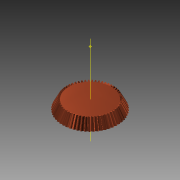
# Autodesk Inventor part: Bevel Gear2
Saved by Autodesk Inventor 2015 (Build 190141000, 141)
## iProperties
Created: 2008-07-23
Part Number: Bevel Gear2
Material: Steel, Mild
Document SubType Name: Modeling
Designer: tangg
Categories: <?xml version="1.0" encoding="UTF-16"?> <MemberInstance><Categories><FamilyTemplate><FamilyTemplateParameter ValueType="xs:double" Id="1" ObjectReferenceKey="da_z" ObjectType="kUserParameterObject"/><FamilyTemplateParameter ValueType="xs:double" Id="2" ObjectReferenceKey="da_b" ObjectType="kUserParameterObject"/><FamilyTemplateParameter ValueType="xs:double" Id="3" ObjectReferenceKey="da_beta" ObjectType="kUserParameterObject"/><FamilyTemplateParameter ValueType="xs:double" Id="4" ObjectReferenceKey="da_dae" ObjectType="kUserParameterObject"/><FamilyTemplateParameter ValueType="xs:double" Id="5" ObjectReferenceKey="da_ve" ObjectType="kUserParameterObject"/><FamilyTemplateParameter ValueType="xs:double" Id="6" ObjectReferenceKey="da_omega" ObjectType="kUserParameterObject"/><FamilyTemplateParameter ValueType="xs:string" Id="7" ObjectReferenceKey="EAIAABAAAAAAHwAAAAAAAIAAAAAAAAAA" ObjectType="83914240" SubObjectId="SurfaceGeometry"/></FamilyTemplate><ParamToTemplateMap><ParamToTemplate CategoryParameter="//CategoryParameter[@InternalName='046C89C9-8512-4d59-83FE-43B91F4F132A']" TemplateParameter="1"/><ParamToTemplate CategoryParameter="//CategoryParameter[@InternalName='2552DF32-E462-4b46-AEBF-C6C7768E72AC']" TemplateParameter="2"/><ParamToTemplate CategoryParameter="//CategoryParameter[@InternalName='C9EE641D-15FC-4fae-A226-E94C4372FDD7']" TemplateParameter="3"/><ParamToTemplate><ParamToTemplate CategoryParameter="//CategoryParameter[@InternalName='00B6519A-459B-49c7-AD84-2E56D39A5744']" ConstantValue="-0.000000"/></ParamToTemplate><ParamToTemplate><ParamToTemplate CategoryParameter="//CategoryParameter[@InternalName='04B31F0E-C7A6-4894-AA32-9629BEFACF47']" ConstantValue="1.000000"/></ParamToTemplate><ParamToTemplate><ParamToTemplate CategoryParameter="//CategoryParameter[@InternalName='43CBEC2E-7847-49e7-A936-2F7889FCB2D9']" ConstantValue="0.200000"/></ParamToTemplate><ParamToTemplate><ParamToTemplate CategoryParameter="//CategoryParameter[@InternalName='B1EFC894-105D-4ebd-86BF-FA20ED196853']" ConstantValue="0.300000"/></ParamToTemplate><ParamToTemplate><ParamToTemplate CategoryParameter="//CategoryParameter[@InternalName='51175063-3D10-4879-93E8-6246FE8B403D']" ConstantValue="2060000000.000000"/></ParamToTemplate><ParamToTemplate><ParamToTemplate CategoryParameter="//CategoryParameter[@InternalName='A3A52E27-4454-46a9-B0BD-C932399B70AF']" ConstantValue="0.300000"/></ParamToTemplate><ParamToTemplate CategoryParameter="//CategoryParameter[@InternalName='2A200944-5A8C-41ca-B96E-8520D2E510F1']" TemplateParameter="4"/><ParamToTemplate><ParamToTemplate CategoryParameter="//CategoryParameter[@InternalName='1A637F62-92C8-44bc-B81F-10802510B579']" ConstantValue="3.389878"/></ParamToTemplate><ParamToTemplate CategoryParameter="//CategoryParameter[@InternalName='B52DD4BE-6863-48fb-BF58-89EF6F9EC65C']" TemplateParameter="5"/><ParamToTemplate><ParamToTemplate CategoryParameter="//CategoryParameter[@InternalName='3956BFF2-84D2-457d-93C2-9B0613DEBA67']" ConstantValue="3.330061"/></ParamToTemplate><ParamToTemplate CategoryParameter="//CategoryParameter[@InternalName='739CFA02-461B-4bf8-8049-181FCAD8B28F']" TemplateParameter="6"/><ParamToTemplate><ParamToTemplate CategoryParameter="//CategoryParameter[@InternalName='A27E999F-E2CE-4481-8A2A-EBF499C4C3C5']" ConstantValue="-0.000000"/></ParamToTemplate><ParamToTemplate><ParamToTemplate CategoryParameter="//CategoryParameter[@InternalName='9E1B4470-B2D3-4ff1-B813-535BB4CDF51A']" ConstantValue="3520000.000000"/></ParamToTemplate><ParamToTemplate><ParamToTemplate CategoryParameter="//CategoryParameter[@InternalName='F8452263-BFF6-458c-9FB1-07C4B99E95CD']" ConstantValue="11400000.000000"/></ParamToTemplate><ParamToTemplate><ParamToTemplate CategoryParameter="//CategoryParameter[@InternalName='3E3BB259-FD49-497f-8171-6EBC954A3479']" ConstantValue="2.000000"/></ParamToTemplate><ParamToTemplate CategoryParameter="//CategoryParameter[@InternalName='27C3BAF2-7550-4e4b-AE2C-0DB134B7D9B7']" TemplateParameter="7"/></ParamToTemplateMap><Category DisplayName="Gear" InternalName="DC85795E-93AB-48d5-8EEE-5A27447B64BD" Mnemonic="Gear"><CategoryParameter DisplayName="z" InternalName="046C89C9-8512-4d59-83FE-43B91F4F132A" Mnemonic="z"/><CategoryParameter DisplayName="b" InternalName="2552DF32-E462-4b46-AEBF-C6C7768E72AC" Mnemonic="b"/><CategoryParameter DisplayName="||b|" InternalName="C9EE641D-15FC-4fae-A226-E94C4372FDD7" Mnemonic="beta"/><CategoryParameter DisplayName="x" InternalName="00B6519A-459B-49c7-AD84-2E56D39A5744" Mnemonic="x"/><CategoryParameter DisplayName="a*" InternalName="04B31F0E-C7A6-4894-AA32-9629BEFACF47" Mnemonic="a"/><CategoryParameter DisplayName="c*" InternalName="43CBEC2E-7847-49e7-A936-2F7889FCB2D9" Mnemonic="c"/><CategoryParameter DisplayName="r|.f|*" InternalName="B1EFC894-105D-4ebd-86BF-FA20ED196853" Mnemonic="rf"/><CategoryParameter DisplayName="E" InternalName="51175063-3D10-4879-93E8-6246FE8B403D" Mnemonic="E"/><CategoryParameter DisplayName="||m|" InternalName="A3A52E27-4454-46a9-B0BD-C932399B70AF" Mnemonic="mi"/><Category DisplayName="BevelGear" InternalName="0C98F69A-0C2B-4791-B2FE-7691BB227E77" Mnemonic="BevelGear"><CategoryParameter DisplayName="d|.ae|" InternalName="2A200944-5A8C-41ca-B96E-8520D2E510F1" Mnemonic="dae"/><CategoryParameter DisplayName="d|.ai|" InternalName="1A637F62-92C8-44bc-B81F-10802510B579" Mnemonic="dai"/><CategoryParameter DisplayName="A|.e|" InternalName="B52DD4BE-6863-48fb-BF58-89EF6F9EC65C" Mnemonic="ve"/><CategoryParameter DisplayName="A|.i|" InternalName="3956BFF2-84D2-457d-93C2-9B0613DEBA67" Mnemonic="vi"/><CategoryParameter DisplayName="||S|" InternalName="739CFA02-461B-4bf8-8049-181FCAD8B28F" Mnemonic="omega"/><CategoryParameter DisplayName="x|.t|" InternalName="A27E999F-E2CE-4481-8A2A-EBF499C4C3C5" Mnemonic="xt"/><CategoryParameter DisplayName="||s||.Flim|" InternalName="9E1B4470-B2D3-4ff1-B813-535BB4CDF51A" Mnemonic="sFlim"/><CategoryParameter DisplayName="||s||.Hlim|" InternalName="F8452263-BFF6-458c-9FB1-07C4B99E95CD" Mnemonic="sHlim"/><CategoryParameter DisplayName="type" InternalName="3E3BB259-FD49-497f-8171-6EBC954A3479" Mnemonic="type"/><CategoryParameter DisplayName="PitchDiameter" InternalName="27C3BAF2-7550-4e4b-AE2C-0DB134B7D9B7" Mnemonic="IDS_PITCHDIAM"/></Category></Category></Categories></MemberInstance>
Mass: 60.9118 g
Surface Area: 34.3074 cm^2
Volume: 7.7496 cm^3
Density: 7.86 g/cm^3
Appearance: Copper - Polished
CustomPartVersion: 1
Author: tangg
Autodesk Inventor part; units mm, degrees
ref_plane "Mesh Plane2" through (0, 0, 0) normal (0.9984815, 0.0550878, 0) x (0, 0, 1)
sketch "Teeth Body Sketch" plane through (0, 0, 0) normal (1, 0, 0) x (0, 1, 0)
  line L0 (0, 0) -> (19.1956, -41.1084) construction
  line L1 (19.1956, -41.1084) -> (20.5787, -40.4311)
  line L2 (20.5787, -40.4311) -> (0, 0) construction
  line L3 (19.95, -40.7389) -> (0, 0) construction
  line L4 (15.8102, -33.8585) -> (16.9494, -33.3006)
  line L5 (19.1956, -41.1084) -> (15.8102, -33.8585)
  line L6 (20.5787, -40.4311) -> (16.9494, -33.3006)
  line L7 (0, -49.33) -> (0, 8.2217) projected
  line L8 (0, -40.7389) -> (20.5787, -40.7389) construction
  dimension "d0" = 39.9
  dimension "d1" = 38.3912
  dimension "d2" = 41.1573
  dimension "d3" = 8
  dimension "d4" = 40.4311
  constraints: 16 end point, 4 point on line, 3 perpendicular, 2 collinear, 1 horizontal alignment, 1 vertical alignment
  measures "d0" diameter of L3.start L7
  measures "d1" diameter of L0.end L7
  measures "d2" diameter of L1.end L7
  measures "d3" distance between parallel lines of L1 L4
  measures "d4" vertical distance of L1.end L0.start
revolve "Teeth Body" add sketch "Teeth Body Sketch" angle 360 about axis through (0, 0, 0) along (0, 0, 1)
ref_plane "Tooth Plane" through (0, 19.1956, -41.1084) normal (0, 0.4398005, -0.8980955) x (-1, 0, 0)
sketch "Start Sketch" plane through (0, 19.1956, -41.1084) normal (0, 0.4398005, -0.8980955) x (-1, 0, 0)
  line L0 (0, -48.8369) -> (0, 14.0347) projected
  arc A0 (-0.2129, -0.1848) -> (-1.1179, 1.9753) centre (-8.2139, -2.2672) ccw
  arc A1 (1.1179, 1.9753) -> (0.2129, -0.1848) centre (8.2139, -2.2672) ccw
  line L1 (-0.2129, -0.1848) -> (0.2129, -0.1848)
  arc A2 (1.1179, 1.9753) -> (-1.1179, 1.9753) centre (0, -21.3737) ccw
  dimension "d7" = 8.2676
  dimension "d8" = 8.2139
  dimension "d9" = 19.1064
  dimension "d57" = 23.3757
  dimension "d58" = 21.1889
  constraints: 6 point on circle, 3 centre point, 3 symmetric about line, 2 end point, 1 coincident, 1 perpendicular, 1 other
  measures "d7" radius of A0
  measures "d8" horizontal distance of point (0, -21.374) A0.centre
  measures "d9" vertical distance of point (0, -21.374) A0.centre
  measures "d57" radius of A2
  measures "d58" distance from line of A2.centre L1
sketch "End Sketch" plane through (0, 15.6433, -33.8545) normal (0, 0.4398005, -0.8980955) x (-1, 0, 0)
  line L0 (0, -44.0369) -> (0, 12.922) projected
  arc A0 (-0.1752, 0.0189) -> (-0.9199, 1.7965) centre (-6.7596, -1.6949) ccw
  arc A1 (0.9199, 1.7965) -> (0.1752, 0.0189) centre (6.7596, -1.6949) ccw
  line L1 (-0.1752, 0.0189) -> (0.1752, 0.0189)
  arc A2 (0.9199, 1.7965) -> (-0.9199, 1.7965) centre (0, -17.4183) ccw
  dimension "d12" = 6.8037
  dimension "d15" = 6.7596
  dimension "d16" = 15.7235
  dimension "d59" = 19.2368
  dimension "d60" = 17.4372
  constraints: 6 point on circle, 3 centre point, 3 symmetric about line, 2 end point, 1 coincident, 1 other
  measures "d12" radius of A0
  measures "d15" horizontal distance of A0.centre point (0, -17.418)
  measures "d16" vertical distance of A0.centre point (0, -17.418)
  measures "d59" radius of A2
  measures "d60" distance from line of A2.centre L1
loft "Loft" cut profiles "Start Sketch", "End Sketch"
pattern_circular "Circular Pattern" count 57 over 360 about axis through (0, 0, 0) along (0, 0, 1) of "Loft"
ref_plane "End Plane" through (0, 15.6433, -33.8545) normal (0, 0.4398005, -0.8980955) x (-1, 0, 0)
sketch3d "3D Sketch Right"
ref_plane "End Plane Right" through (-0.668, 16.3841, -33.485) normal (0.017917, -0.4394354, 0.8980955) x (0.9991698, 0.0407389, 0)
sketch "End Sketch Right" plane through (-0.668, 16.3841, -33.485) normal (0.017917, -0.4394354, 0.8980955) x (0.9991698, 0.0407389, 0)
  arc A0 (-0.1752, -0.8211) -> (-0.9199, 0.9565) centre (-6.7596, -2.5349) ccw
  line L0 (0, -22.7985) -> (0, 5.5231) projected
  arc A1 (0.9199, 0.9565) -> (0.1752, -0.8211) centre (6.7596, -2.5349) ccw
  line L1 (-0.1752, -0.8211) -> (0.1752, -0.8211)
  arc A2 (0.9199, 0.9565) -> (-0.9199, 0.9565) centre (0, -18.2583) ccw
  dimension "d70" = 6.7596
  dimension "d71" = 15.7235
  dimension "d72" = 6.8037
  dimension "d73" = 17.4372
  dimension "d74" = 19.2368
  constraints: 6 point on circle, 3 centre point, 3 symmetric about line, 2 end point, 1 coincident, 1 perpendicular, 1 other
  measures "d70" horizontal distance of A2.centre A0.centre
  measures "d71" vertical distance of point (0, -18.258) A0.centre
  measures "d72" radius of A0
  measures "d73" distance from line of point (0, -18.258) L1
  measures "d74" radius of A2
feature "Loft Right" [suppressed]
pattern_circular "Circular Pattern Right" [suppressed]
sketch3d "3D Sketch Left"
ref_plane "End Plane Left" through (0.6593, 16.3841, -33.4842) normal (-0.0176822, -0.4394457, 0.8980951) x (0.9991914, -0.0402051, 0)
sketch "End Sketch Left" plane through (0.6593, 16.3841, -33.4842) normal (-0.0176822, -0.4394457, 0.8980951) x (0.9991914, -0.0402051, 0)
  line L0 (0, -37.7502) -> (0, 8.8653) projected
  arc A0 (-0.1752, -0.8212) -> (-0.9199, 0.9564) centre (-6.7596, -2.5349) ccw
  arc A1 (0.9199, 0.9564) -> (0.1752, -0.8212) centre (6.7596, -2.5349) ccw
  line L1 (-0.1752, -0.8212) -> (0.1752, -0.8212)
  ellipse E0 centre (0, -14.6457) end of major axis (16.9494, -14.6457) minor radius 15.2222 projected
  arc A2 (0.9199, 0.9564) -> (-0.9199, 0.9564) centre (0, -18.2584) ccw
  dimension "d56" = 15.2222
  dimension "d30" = 6.8037
  dimension "d31" = 6.7596
  dimension "d32" = 15.7235
  dimension "d61" = 19.2368
  dimension "d62" = 17.4372
  constraints: 6 point on circle, 3 centre point, 3 symmetric about line, 2 end point, 1 coincident, 2 other
  measures "d30" radius of A0
  measures "d31" horizontal distance of point (0, -18.258) A0.centre
  measures "d32" vertical distance of A0.centre point (0, -18.258)
  measures "d61" radius of A2
  measures "d62" distance from line of point (0, -18.258) L1
feature "Loft Left" [suppressed]
pattern_circular "Circular Pattern Left" [suppressed]
sketch "Body Sketch" plane through (0, 0, 0) normal (1, 0, 0) x (0, 1, 0)
  line L0 (0, -42.5584) -> (0, -32.4085) projected
  line L1 (19.1956, -41.1084) -> (15.8102, -33.8585) projected
  line L2 (15.8102, -33.8585) -> (0, -33.8585)
  line L3 (19.1956, -41.1084) -> (0, -41.1084)
  constraints: 4 end point, 2 perpendicular, 2 point on line
revolve "Fix Body" add sketch "Body Sketch" angle 360 about axis through (0, 0, 0) along (0, 0, 1)
sketch "Sketch6" plane through (0, 0, 0) normal (1, 0, 0) x (0, 1, 0)
  line L0 (19.95, -40.7389) -> (0, 0) projected
  line L1 (0, -48.8867) -> (0, 8.1478) projected
surface revolve "Pitch Diameter" sketch "Sketch6" angle 360 about axis through (0, 0, 0) along (0, 0, 1) shown no curves L0
equation "\"d0\" = da_de"
equation "\"d1\" = da_dfe"
equation "\"d2\" = da_dae"
equation "\"d3\" = da_b"
equation "\"d4\" = da_ve"
equation "\"d7\" = fd_rr"
equation "\"d8\" = fd_x"
equation "\"d9\" = fd_y"
equation "\"d57\" = 0.5 * fd_dva + 0.3 * da_he"
equation "\"d58\" = 0.5 * fd_dva - 1.12 * da_he"
equation "\"da_teethtype\" = 0"
equation "\"da_b\" = 8"
equation "\"da_de\" = 39.9"
equation "\"da_dae\" = 41.15733"
equation "\"da_dfe\" = 38.3912"
equation "\"da_le\" = 45.36148"
equation "\"da_omega\" = 45deg"
equation "\"da_beta\" = 0"
equation "\"da_delta\" = 26.091152deg"
equation "\"da_alpha\" = 20deg"
equation "\"da_he\" = 1.54"
equation "\"da_ve\" = 40.43108"
equation "\"da_zv\" = 63.467638"
equation "\"fd_loft\" = da_b + 0.05 * da_he"
equation "\"fd_x\" = fd_x1 + fd_x2"
equation "\"fd_y\" = fd_y1 - fd_y2"
equation "\"fd_dd\" = fd_dva - 0.6 * da_he"
equation "\"da_dvw\" = 44.42735"
equation "\"d11\" = -fd_loft"
equation "\"da_dm\" = 36.3816"
equation "\"da_x\" = 0"
equation "\"da_m\" = 0.7"
equation "\"fd_rr\" = 8.26757"
equation "\"fd_dva\" = 45.827346"
equation "\"fd_x1\" = 0.549723"
equation "\"fd_x2\" = 7.664202"
equation "\"fd_y1\" = 22.20687"
equation "\"fd_y2\" = 3.10044"
body "Solid1"
body "Srf1"
